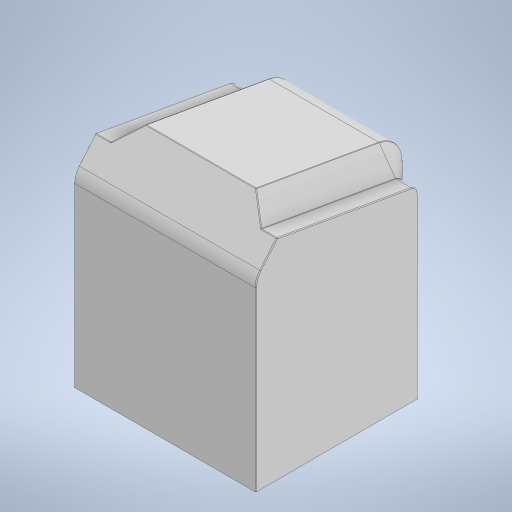
# Autodesk Inventor part: Printer Envelope Study
Saved by Autodesk Inventor 2024 (Build 280153000, 153)
## iProperties
Created: 2024-07-22
Part Number: Printer Envelope Study
Material: Generic
Document SubType Name: Modeling
Designer: Ishaan
Density: 1 g/cm^3
Appearance: Default
Author: Ishaan
Autodesk Inventor part; units mm, degrees
ref_plane "YZ Plane" through (0, 0, 0) normal (1, 0, 0) x (0, 1, 0)
ref_plane "XZ Plane" through (0, 0, 0) normal (0, 1, 0) x (-1, 0, 0)
sketch "Sketch1" plane through (0, 0, 0) normal (0, 0, 1) x (1, 0, 0)
  line L0 (230, -205) -> (-230, -205)
  line L1 (-230, -205) -> (-230, 205)
  line L2 (-230, 205) -> (230, 205)
  line L3 (230, 205) -> (230, -205)
  line L4 (230, -205) -> (-230, 205) construction
  line L5 (-230, -205) -> (230, 205) construction
  line L6 (-190, 205) -> (-139.1421, 255.8579)
  line L7 (-139.1421, 255.8579) -> (139.1421, 255.8579)
  line L8 (139.1421, 255.8579) -> (190, 205)
  line L9 (139.1421, 255.8579) -> (135.0218, 245.9106) construction
  line L10 (135, 255.8579) -> (135, 245.8579) construction
  line L11 (230, 205) -> (190, 205)
  line L12 (190, 205) -> (190, 165)
  line L13 (190, 165) -> (230, 165)
  line L14 (230, 165) -> (230, 205)
  line L15 (-150, 105) -> (150, 105)
  line L16 (150, 105) -> (150, -145)
  line L17 (150, -145) -> (-150, -145)
  line L18 (-150, -145) -> (-150, 105)
  line L19 (-230, -205) -> (-190, -205)
  line L20 (-190, -205) -> (-190, -165)
  line L21 (-190, -165) -> (-230, -165)
  line L22 (-230, -165) -> (-230, -205)
  line L23 (230, -205) -> (190, -205)
  line L24 (190, -205) -> (190, -165)
  line L25 (190, -165) -> (230, -165)
  line L26 (230, -165) -> (230, -205)
  line L27 (-230, 205) -> (-190, 205)
  line L28 (-190, 205) -> (-190, 165)
  line L29 (-190, 165) -> (-230, 165)
  line L30 (-230, 165) -> (-230, 205)
  line L31 (-40, 205) -> (40, 205)
  line L32 (40, 205) -> (40, 165)
  line L33 (40, 165) -> (-40, 165)
  line L34 (-40, 165) -> (-40, 205)
  line L35 (125, 255.8579) -> (135, 255.8579)
  line L36 (135, 255.8579) -> (135, 235.8579)
  line L37 (135, 235.8579) -> (125, 235.8579)
  line L38 (125, 235.8579) -> (125, 255.8579)
  line L39 (149.1421, 245.8579) -> (142.0711, 252.9289)
  line L40 (142.0711, 252.9289) -> (127.9289, 238.7868)
  line L41 (127.9289, 238.7868) -> (135, 231.7157)
  line L42 (135, 231.7157) -> (149.1421, 245.8579)
  line L43 (135, 205) -> (132, 205)
  line L44 (132, 205) -> (132, 231)
  line L45 (132, 231) -> (135, 231)
  line L46 (135, 231) -> (135, 205)
  line L47 (135, 205) -> (95, 205)
  line L48 (95, 205) -> (95, 185)
  line L49 (95, 185) -> (135, 185)
  line L50 (135, 185) -> (135, 205)
  line L51 (-222, 75) -> (-132, 75)
  line L52 (-132, 75) -> (-132, -145)
  line L53 (-132, -145) -> (-222, -145)
  line L54 (-222, -145) -> (-222, 75)
  point P0 (0, 0)
  point P1 (0, 105)
  point P2 (0, 205)
  dimension "d0" = 460
  dimension "d1" = 410
  dimension "d2" = 40
  dimension "d3" = 40
  dimension "d4" = 135
  dimension "d5" = 135
  dimension "d30" = 67.5
  dimension "d32" = 10
  dimension "d34" = 50.8579
  dimension "d35" = 40
  dimension "d36" = 40
  dimension "d37" = 300
  dimension "d38" = 250
  dimension "d39" = 60
  dimension "d40" = 40
  dimension "d41" = 40
  dimension "d42" = 40
  dimension "d43" = 40
  dimension "d44" = 40
  dimension "d45" = 40
  dimension "d46" = 80
  dimension "d47" = 40
  dimension "d48" = 10
  dimension "d50" = 10
  dimension "d51" = 3
  dimension "d52" = 26
  dimension "d53" = 40
  dimension "d54" = 20
  dimension "d55" = 55
  dimension "d56" = 105
  dimension "d57" = 90
  dimension "d58" = 220
  dimension "d59" = 8
  dimension "d60" = 20
  dimension "d61" = 55
  constraints: 110 end point, 24 parallel, 12 horizontal, 12 perpendicular, 8 point on line, 7 midpoint, 1 vertical, 1 vertical alignment
  measures "d0" distance of L1.end L2.end
  measures "d1" distance of L0.end L1.end
  measures "d2" distance from line of L3 L8.end
  measures "d3" distance from line of L6.start L1
  measures "d4" angle of L7 L6
  measures "d5" angle of L8 L7
  measures "d30" angle of L9 L7
  measures "d32" distance of L10.end L10.start
  measures "d34" distance between parallel lines of L2 L7
  measures "d35" distance of L13.end L12.end
  measures "d36" distance of L12.end L11.end
  measures "d37" distance of L16.end L17.end
  measures "d38" distance of L15.end L16.end
  measures "d39" distance between parallel lines of L0 L17
  measures "d40" distance of L21.end L20.end
  measures "d41" distance of L20.end L19.end
  measures "d42" distance of L24.end L25.end
  measures "d43" distance of L23.end L24.end
  measures "d44" distance of L28.end L29.end
  measures "d45" distance of L27.end L28.end
  measures "d46" distance of L32.end L33.end
  measures "d47" distance of L31.end L32.end
  measures "d48" distance of L36.end L37.end
  measures "d50" distance of L40.end L41.end
  measures "d51" distance of L44.end L45.end
  measures "d52" distance of L45.end L43.start
  measures "d53" distance of L49.end L48.end
  measures "d54" distance of L48.end L47.end
  measures "d55" distance between parallel lines of L48 L32
  measures "d56" distance between parallel lines of L3 L38
  measures "d57" distance of L52.end L53.end
  measures "d58" distance of L51.end L52.end
  measures "d59" distance between parallel lines of L1 L54
  measures "d60" distance between parallel lines of L21 L53
  measures "d61" distance between parallel lines of L12 L50
extrude "Extrusion1" add sketch "Sketch1" along normal blind 450 contours L0 L24 L25 L3 | L0 L20 L21 L1 L29 L28 L2 L34 L33 L32 L48 L49 L50 L12 L13 L3 L25 L24 | L0 L1 L21 L20 | L13 L12 L2 L3 | L2 L46 L45 L44 L6 L7 L38 L37 L41 L42 L8 | L1 L2 L28 L29 | L50 L49 L48 L2 | L2 L44 L45 L46 | L42 L41 L37 L36 L40 L8 | L40 L36 L7 L8 | L40 L41 L37 L38 L7 L36 | L36 L37 L41 L40 | L2 L32 L33 L34 | L15 L16 L17 L52 L51 L18 | L51 L52 L17 L18 | L18 L53 L54 L51
sketch "Sketch2" plane through (0, 0, 450) normal (0, 0, 1) x (1, 0, 0)
  line L0 (-139.1421, 255.8579) -> (-190, 205) projected
  line L1 (-190, 205) -> (-230, 205) projected
  line L2 (-230, 205) -> (-230, -205) projected
  line L3 (-230, -205) -> (230, -205) projected
  line L4 (230, -205) -> (230, 205) projected
  line L5 (230, 205) -> (190, 205) projected
  line L6 (190, 205) -> (139.1421, 255.8579) projected
  line L7 (139.1421, 255.8579) -> (-139.1421, 255.8579) projected
  line L8 (230, 185) -> (-230, 185)
  point P0 (0, 0)
  dimension "d9" = 20
  constraints: 2 end point, 2 point on line
  measures "d9" distance between parallel lines of L8 L1
revolve "Revolution1" add sketch "Sketch2" angle 80 about axis through (230, 185, 450) along (1, 0, 0) contours L7 L6 L5 L4 L8 L2 L1 L0
sketch "Sketch3" plane through (-230, 185, 450) normal (0, -0.9848078, 0.1736482) x (1, 0, 0)
  line L0 (0, 20) -> (0, 0) projected
  line L1 (460, 0) -> (0, 0) projected
  line L2 (460, 0) -> (460, 20) projected
  line L3 (460, 20) -> (420, 20) projected
  line L4 (420, 20) -> (369.1421, 70.8579) projected
  line L5 (369.1421, 70.8579) -> (90.8579, 70.8579) projected
  line L6 (90.8579, 70.8579) -> (40, 20) projected
  line L7 (40, 20) -> (0, 20) projected
  point P0 (230, -475.2884)
ref_plane "Work Plane4" through (-230, -212.6604, 456.4279) normal (0, 0.7660444, -0.6427876) x (1, 0, 0)
ref_plane "Work Plane3" through (-230, -205, 450) normal (0, 0.7660444, -0.6427876) x (1, 0, 0)
extrude "Extrusion5" add sketch "Sketch3" along normal up to surface surface through (-230, -212.6604, 456.4279) normal (0, 0.7660444, -0.6427876)
sketch "Sketch6" plane through (-230, -205, 0) normal (-1, 0, 0) x (0, 0, 1)
  line L0 (0, 410) -> (0, 0) projected
  line L1 (0, 0) -> (450, 0) projected
  line L2 (450, 390) -> (450, 0) projected
  line L3 (450, 390) -> (511.9094, 38.8941) projected
  line L4 (529.6005, 53.7387) -> (511.9094, 38.8941) projected
  line L5 (469.6962, 393.473) -> (529.6005, 53.7387) projected
  arc A0 (469.6962, 393.473) -> (450, 410) centre (450, 390) ccw projected
  line L6 (0, 410) -> (450, 410) projected
  line L7 (511.9094, 38.8941) -> (465.5572, 0)
  line L8 (465.5572, 0) -> (450, 0)
  point P0 (0, 205)
  constraints: 4 end point, 1 collinear, 1 horizontal
extrude "Extrusion6" add sketch "Sketch6" against normal up to surface (460 mm away) contours L2 L3 L7 L8
fillet "Fillet1" radius 50 1 edges at (0, -205, 465.5572)
fillet "Fillet3" radius 2 6 edges at (-190, 200.3209, 462.8558) (-190, 205, 225) (-190, 18.6058, 499.6483) (190, 200.3209, 462.8558) (190, 205, 225) (190, 18.6058, 499.6483)
fillet "Fillet4" radius 2 13 edges at (0, -113.5133, 574.5869) (-139.1421, 239.2803, 495.5466) (-139.1421, 255.8579, 225) (-139.1421, 41.8955, 547.1841) (-190.0631, -151.1483, 529.7351) (-210.4142, -151.2613, 529.6005) (-164.2782, -132.1699, 552.3528) (190.0631, -151.1483, 529.7351) (210.4142, -151.2613, 529.6005) (164.2782, -132.1699, 552.3528) (139.1421, 239.2803, 495.5466) (139.1421, 255.8579, 225) (139.1421, 41.8955, 547.1841)
fillet "Fillet5" radius 2 14 edges at (-230, -151.1555, 529.3097) (-230, 19.1744, 499.5481) (-230, 200.3209, 462.8558) (-230, 205, 225) (-230, -201.9846, 464.4597) (-230, -205, 223.6794) (-230, -172.6529, 504.107) (230, -151.1555, 529.3097) (230, 19.1744, 499.5481) (230, 200.3209, 462.8558) (230, 205, 225) (230, -201.9846, 464.4597) (230, -205, 223.6794) (230, -172.6529, 504.107)
equation "\"d30\" = 0.5 * d5"
body "Solid1"
